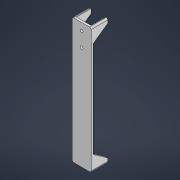
# Autodesk Inventor part: Z Drill Template
Saved by Autodesk Inventor 2022 (Build 260153000, 153)
## iProperties
Created: 2022-02-13
Part Number: Z Drill Template
Material: Generic
Document SubType Name: Modeling
Designer: nicol
Density: 1 g/cm^3
Appearance: Default
Author: nicol
Autodesk Inventor part; units mm, degrees
ref_plane "YZ Plane" through (0, 0, 0) normal (1, 0, 0) x (0, 1, 0)
ref_plane "XZ Plane" through (0, 0, 0) normal (0, 1, 0) x (-1, 0, 0)
ref_plane "XY Plane" through (0, 0, 0) normal (0, 0, 1) x (1, 0, 0)
sketch "Sketch1" plane through (0, 0, 0) normal (0, 0, 1) x (1, 0, 0)
  line L0 (0, 0) -> (20, 0)
  line L1 (20, 0) -> (20, 172.5)
  line L2 (20, 172.5) -> (0, 172.5)
  line L3 (0, 172.5) -> (0, 0)
  line L4 (0, 0) -> (0, 172.5)
  line L5 (0, 172.5) -> (-3, 172.5)
  line L6 (-3, 172.5) -> (-3, 0)
  line L7 (-3, 0) -> (0, 0)
  line L8 (20, 172.5) -> (20, 0)
  line L9 (20, 0) -> (23, 0)
  line L10 (23, 0) -> (23, 172.5)
  line L11 (23, 172.5) -> (20, 172.5)
  line L12 (23, 20) -> (-3, 20)
  point P0 (0, 20)
  point P1 (20, 20)
  dimension "d0" = 20
  dimension "d1" = 172.5
  dimension "d2" = 3
  dimension "d3" = 3
  dimension "d6" = 20
  constraints: 26 end point, 8 equal length, 4 perpendicular, 2 point on line, 1 horizontal
  measures "d0" distance of L2.end L1.end
  measures "d1" distance of L1.end L0.end
  measures "d2" distance of L5.end L2.end
  measures "d3" distance of L9.end L0.end
  measures "d6" distance between parallel lines of L0 L12
extrude "Extrusion1" add sketch "Sketch1" along normal blind 3
extrude "Extrusion2" add sketch "Sketch1" against normal blind 20 contours L7 L6 L12 L3 | L1 L12 L10 L9
chamfer "Chamfer1" distance 20 angle 35 1 edges at (-1.5, 20, -20) measured on face at (-1.5, 20, -19.5)
chamfer "Chamfer2" distance 20 angle 35 1 edges at (21.5, 20, -20) measured on face at (21.5, 20, -19.5)
sketch "Sketch2" plane through (0, 0, 3) normal (0, 0, 1) x (1, 0, 0)
  circle A0 centre (10, 162.5) radius 2 projected
  circle A1 centre (10, 142.5) radius 2 projected
  point P0 (0, 0)
extrude "Extrusion3" cut sketch "Sketch2" against normal through all
ref_plane "Work Plane2" through (-3, 86.25, 0) normal (0, 1, 0) x (1, 0, 0)
mirror "Mirror2" about plane through (-3, 86.25, 0) normal (0, 1, 0) of "Extrusion2", "Chamfer1", "Chamfer2"
fillet "Fillet1" radius 2 4 edges at (23, 0, -8.5) (-3, 0, -8.5) (23, 172.5, -8.5) (-3, 172.5, -8.5)
body "Solid1"
